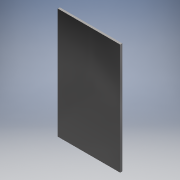
# Autodesk Inventor part: LeftRightInner
Saved by Autodesk Inventor 2017 (Build 210142000, 142)
## iProperties
Created: 2016-12-13
Part Number: LeftRightInner
Material: Steel, Mild
Document SubType Name: Sheet Metal
Designer: Robert.Chapman
Density: 7.85 g/cm^3
Sheet Metal Rule: Default
Appearance: Semi-Polished
Mass: 1543.66 g
Surface Area: 865.482 cm^2
Volume: 196.645 cm^3
Author: Robert.Chapman
Autodesk Inventor part; units mm, degrees
ref_plane "YZ Plane" through (0, 0, 0) normal (1, 0, 0) x (0, 1, 0)
ref_plane "XZ Plane" through (0, 0, 0) normal (0, 1, 0) x (-1, 0, 0)
ref_plane "XY Plane" through (0, 0, 0) normal (0, 0, 1) x (1, 0, 0)
sketch "Sketch3" plane through (0, 0, 0) normal (0, 0, 1) x (1, 0, 0)
  line L0 (-76.2, -127) -> (76.2, -127)
  line L1 (76.2, -127) -> (76.2, 127)
  line L2 (76.2, 127) -> (-76.2, 127)
  line L3 (-76.2, 127) -> (-76.2, -127)
  line L4 (-76.2, -127) -> (76.2, 127) construction
  line L5 (76.2, -127) -> (-76.2, 127) construction
  point P0 (0, 0)
  dimension "d3" = 152.4
  dimension "d4" = 254
  measures "d3" distance of L1.end L2.end
  measures "d4" distance of L2.end L0.start
extrude "Plate2" add sketch "Sketch3" along normal blind 4.7625
equation "\"BendRadius\" = Thickness"
equation "\"BendReliefWidth\" = Thickness"
equation "\"BendReliefDepth\" = 0.5 * Thickness"
equation "\"CornerReliefSize\" = 4 * Thickness"
equation "\"MinimumRemnant\" = 2 * Thickness"
equation "\"TransitionRadius\" = BendRadius"
equation "\"JacobiRadiusSize\" = BendRadius"
equation "\"GapSize\" = Thickness"
equation "\"d2\" = BendRadius"
equation "\"d5\" = BendRadius"
equation "\"Thickness\" = 4.7625"
body "Solid2"
